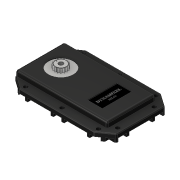
# Autodesk Inventor part: Depan
Saved by Autodesk Inventor 2019 (Build 230136000, 136)
## iProperties
Created: 2021-08-24
Part Number: Depan
Material: Generic
Document SubType Name: Modeling
Designer: user
Density: 1 g/cm^3
Appearance: Glossy - Black
Author: user
Autodesk Inventor part; units mm, degrees
(part 1 of 2)
ref_plane "YZ Plane" through (0, 0, 0) normal (1, 0, 0) x (0, 1, 0)
ref_plane "XZ Plane" through (0, 0, 0) normal (0, 1, 0) x (-1, 0, 0)
ref_plane "XY Plane" through (0, 0, 0) normal (0, 0, 1) x (1, 0, 0)
sketch "Sketch1" plane through (0, 0, 0) normal (0, 1, 0) x (-1, 0, 0)
  line L0 (30.55, -20.1) -> (-30.55, -20.1)
  line L1 (-30.55, -20.1) -> (-30.55, 20.1)
  line L2 (-30.55, 20.1) -> (30.55, 20.1)
  line L3 (30.55, 20.1) -> (30.55, -20.1)
  line L4 (30.55, -20.1) -> (-30.55, 20.1) construction
  line L5 (-30.55, -20.1) -> (30.55, 20.1) construction
  circle A0 centre (17.55, 0) radius 5
  circle A1 centre (17.55, 0) radius 14
  line L6 (-24.95, -14.5) -> (30.55, -14.5)
  line L7 (30.55, -14.5) -> (30.55, 14.5)
  line L8 (30.55, 14.5) -> (-24.95, 14.5)
  line L9 (-24.95, 14.5) -> (-24.95, -14.5)
  line L10 (-24.95, -14.5) -> (30.55, 14.5) construction
  line L11 (30.55, -14.5) -> (-24.95, 14.5) construction
  circle A2 centre (21.55, 17.3) radius 1.25
  circle A3 centre (21.55, -17.3) radius 1.25
  circle A4 centre (-0.45, 17.3) radius 1.25
  circle A5 centre (-0.45, -17.3) radius 1.25
  circle A6 centre (-22.45, 17.3) radius 1.25
  circle A7 centre (-22.45, -17.3) radius 1.25
  circle A8 centre (-27.75, -11) radius 1.25
  circle A9 centre (-27.75, 11) radius 1.25
  line L12 (30.55, 14.5) -> (22.55, 20.1)
  line L13 (-30.55, 14.5) -> (-22.55, 20.1)
  line L14 (30.55, -14.5) -> (22.55, -20.1)
  line L15 (-30.55, -14.5) -> (-22.55, -20.1)
  point P0 (0, 0)
  point P1 (2.8, 0)
  point P2 (30.55, 0)
  dimension "d0" = 61.1
  dimension "d1" = 40.2
  dimension "d2" = 10
  dimension "d3" = 13
  dimension "d4" = 28
  dimension "d5" = 55.5
  dimension "d6" = 29
  dimension "d9" = 4
  dimension "d10" = 2.8
  dimension "d13" = 34.6
  dimension "d16" = 22
  dimension "d20" = 2.8
  dimension "d23" = 22
  dimension "d24" = 11
  dimension "d25" = 8
  constraints: 32 end point, 10 centre point, 6 point on line, 5 midpoint, 4 parallel, 3 horizontal, 2 perpendicular, 1 coincident, 1 vertical, 10 other
  measures "d0" distance of L1.end L2.end
  measures "d1" distance of L0.end L1.end
  measures "d2" diameter of A0
  measures "d3" distance from line of L3 A0.centre
  measures "d4" diameter of A1
  measures "d5" distance of L8.end L7.end
  measures "d6" distance of L7.end L6.end
  measures "d9" horizontal distance of A2.centre A0.centre
  measures "d10" distance from line of L2 A2.centre
  measures "d13" distance of A2.centre A3.centre
  measures "d16" distance of A2.centre A4.centre
  measures "d20" distance from line of L1 A8.centre
  measures "d23" distance of A9.centre A8.centre
  measures "d24" vertical distance of A8.centre point (0, 0)
  measures "d25" distance of L2.end L12.end
extrude "Extrusion1" add sketch "Sketch1" against normal blind 4.6 contours L0 L15 L1 L13 L2 L12 L8 L9 L6 L14 | L6 L9 L8 L3 A1 | A1 L3 | A0 picked at (27.8833, 0)
sketch "Sketch2" plane through (0, 0, 0) normal (0, 1, 0) x (1, 0, 0)
  line L0 (-30.55, 20.1) -> (30.55, -20.1) construction
  line L1 (30.55, 20.1) -> (-30.55, -20.1) construction
  circle A0 centre (-17.55, 0) radius 1.25
  circle A1 centre (-17.55, 0) radius 14
  line L2 (24.95, 14.5) -> (-30.55, 14.5)
  line L3 (-30.55, 14.5) -> (-30.55, -14.5)
  line L4 (-30.55, -14.5) -> (24.95, -14.5)
  line L5 (24.95, -14.5) -> (24.95, 14.5)
  line L6 (24.95, 14.5) -> (-30.55, -14.5) construction
  line L7 (-30.55, 14.5) -> (24.95, -14.5) construction
  point P0 (0, 0)
  point P1 (0, 0)
  point P2 (-2.8, 0)
  point P3 (-30.55, 0)
  dimension "d33" = 2.5
  dimension "d34" = 28
  dimension "d35" = 55.5
  dimension "d36" = 29
  constraints: 16 end point, 5 midpoint, 2 centre point, 2 parallel, 1 coincident, 1 perpendicular
  measures "d33" diameter of A0
  measures "d34" diameter of A1
  measures "d35" distance of L7.end L3.end
  measures "d36" distance of L3.end L3.start
extrude "Extrusion2" add sketch "Sketch2" along normal blind 3.5 contours A1 L3 | A1 L3 L2 L5 L4 picked at (-26.6333, 0)
fillet "Fillet1" radius 1 15 edges at (30.55, -2.3, -14.5) (22.55, -2.3, -20.1) (30.55, -2.3, 14.5) (22.55, -2.3, 20.1) (-22.55, -2.3, 20.1) (-22.55, -2.3, -20.1) (24.95, 1.75, -14.5) (24.95, 1.75, 14.5) (-30.55, 1.75, 14.5) (-30.55, 1.75, -14.5) (-30.55, -2.3, -14.5) (-30.55, -2.3, 14.5) (24.95, 3.5, 0) (-2.8, 3.5, -14.5) (-2.8, 3.5, 14.5)
fillet "Fillet2" radius 0.5 17 edges at (22.5354, 0, 20.0537) (26.4659, 0, 17.3589) (30.437, 0, 14.4412) (30.55, 0, 0) (30.437, 0, -14.4412) (26.4659, 0, -17.3589) (22.5354, 0, -20.0537) (0, 0, -20.1) (-22.5354, 0, -20.0537) (-26.4659, 0, -17.3589) (-30.437, 0, -14.4412) (-30.55, 0, -13.7397) (-22.5354, 0, 20.0537) (-26.4659, 0, 17.3589) (-30.437, 0, 14.4412) (-30.55, 0, 13.7397) (0, 0, 20.1)
fillet "Fillet3" radius 2 3 edges at (-30.2571, 3.2071, 14.2071) (-30.2571, 3.2071, -14.2071) (-30.55, 3.5, 0)
sketch "Sketch4" plane through (0, 3.5, 0) normal (0, 1, 0) x (1, 0, 0)
  circle A0 centre (-17.55, 0) radius 1.25 projected
  circle A1 centre (-17.55, 0) radius 7.5
  line L0 (7.45, -9) -> (16.45, -9)
  line L1 (16.45, -9) -> (16.45, 9)
  line L2 (16.45, 9) -> (7.45, 9)
  line L3 (7.45, 9) -> (7.45, -9)
  line L4 (7.45, -9) -> (16.45, 9) construction
  line L5 (16.45, -9) -> (7.45, 9) construction
  point P0 (0, 0)
  point P1 (11.95, 0)
  dimension "d53" = 15
  dimension "d63" = 9
  dimension "d64" = 18
  dimension "d65" = 25
  constraints: 12 end point, 2 midpoint, 2 parallel, 1 centre point, 1 coincident, 1 horizontal, 1 perpendicular
  measures "d53" diameter of A1
  measures "d63" distance of L2.end L1.end
  measures "d64" distance of L1.end L0.end
  measures "d65" distance from line of L3 A1.centre
extrude "Extrusion3" cut sketch "Sketch4" against normal blind 0.5
sketch "Sketch5" plane through (-17.55, 3, 0) normal (0, 1, 0) x (1, 0, 0)
  line L0 (-1.8334, 2.6835) -> (-2.7146, 2.7146)
  line L1 (-2.7146, 2.7146) -> (-2.6835, 1.8334)
  arc A0 (-1.8334, 2.6835) -> (-2.6835, 1.8334) centre (0, 0) ccw
  line L2 (-0.667, 3.1808) -> (-1.4691, 3.5467)
  line L3 (-1.4691, 3.5467) -> (-1.7776, 2.7208)
  arc A1 (-0.667, 3.1808) -> (-1.7776, 2.7208) centre (0, 0) ccw
  arc A2 (0.6011, 3.1939) -> (-0.6011, 3.1939) centre (0, 0) ccw
  line L4 (0.6011, 3.1939) -> (0, 3.839)
  line L5 (0, 3.839) -> (-0.6011, 3.1939)
  arc A3 (0.6011, 3.1939) -> (-0.6011, 3.1939) centre (0, 0) ccw
  line L6 (1.7776, 2.7208) -> (1.4691, 3.5467)
  line L7 (1.4691, 3.5467) -> (0.667, 3.1808)
  arc A4 (1.7776, 2.7208) -> (0.667, 3.1808) centre (0, 0) ccw
  line L8 (2.6835, 1.8334) -> (2.7146, 2.7146)
  line L9 (2.7146, 2.7146) -> (1.8334, 2.6835)
  arc A5 (2.6835, 1.8334) -> (1.8334, 2.6835) centre (0, 0) ccw
  line L10 (3.1808, 0.667) -> (3.5467, 1.4691)
  line L11 (3.5467, 1.4691) -> (2.7208, 1.7776)
  arc A6 (3.1808, 0.667) -> (2.7208, 1.7776) centre (0, 0) ccw
  line L12 (3.1939, -0.6011) -> (3.839, 0)
  line L13 (3.839, 0) -> (3.1939, 0.6011)
  arc A7 (3.1939, -0.6011) -> (3.1939, 0.6011) centre (0, 0) ccw
  line L14 (2.7208, -1.7776) -> (3.5467, -1.4691)
  line L15 (3.5467, -1.4691) -> (3.1808, -0.667)
  arc A8 (2.7208, -1.7776) -> (3.1808, -0.667) centre (0, 0) ccw
  line L16 (1.8334, -2.6835) -> (2.7146, -2.7146)
  line L17 (2.7146, -2.7146) -> (2.6835, -1.8334)
  arc A9 (1.8334, -2.6835) -> (2.6835, -1.8334) centre (0, 0) ccw
  line L18 (0.667, -3.1808) -> (1.4691, -3.5467)
  line L19 (1.4691, -3.5467) -> (1.7776, -2.7208)
  arc A10 (0.667, -3.1808) -> (1.7776, -2.7208) centre (0, 0) ccw
  line L20 (-0.6011, -3.1939) -> (0, -3.839)
  line L21 (0, -3.839) -> (0.6011, -3.1939)
  arc A11 (-0.6011, -3.1939) -> (0.6011, -3.1939) centre (0, 0) ccw
  line L22 (-1.7776, -2.7208) -> (-1.4691, -3.5467)
  line L23 (-1.4691, -3.5467) -> (-0.667, -3.1808)
  arc A12 (-1.7776, -2.7208) -> (-0.667, -3.1808) centre (0, 0) ccw
  line L24 (-2.6835, -1.8334) -> (-2.7146, -2.7146)
  line L25 (-2.7146, -2.7146) -> (-1.8334, -2.6835)
  arc A13 (-2.6835, -1.8334) -> (-1.8334, -2.6835) centre (0, 0) ccw
  line L26 (-3.1808, -0.667) -> (-3.5467, -1.4691)
  line L27 (-3.5467, -1.4691) -> (-2.7208, -1.7776)
  arc A14 (-3.1808, -0.667) -> (-2.7208, -1.7776) centre (0, 0) ccw
  line L28 (-3.1939, 0.6011) -> (-3.839, 0)
  line L29 (-3.839, 0) -> (-3.1939, -0.6011)
  arc A15 (-3.1939, 0.6011) -> (-3.1939, -0.6011) centre (0, 0) ccw
  line L30 (-2.7208, 1.7776) -> (-3.5467, 1.4691)
  line L31 (-3.5467, 1.4691) -> (-3.1808, 0.667)
  arc A16 (-2.7208, 1.7776) -> (-3.1808, 0.667) centre (0, 0) ccw
  circle A17 centre (0, 0) radius 3.25
  circle A18 centre (0, 0) radius 1.25
  point P0 (17.55, 0)
  constraints: 64 end point, 34 point on circle, 19 centre point
extrude "Extrusion4" add sketch "Sketch5" along normal blind 2.5 contours A17 A1 A2 A4 A5 A6 A7 A8 A9 A10 A11 A12 A13 A14 A15 A16 A0
sketch "Sketch6" plane through (-17.55, 3, 0) normal (0, 1, 0) x (1, 0, 0)
  line L0 (-1.8334, 2.6835) -> (-2.7146, 2.7146)
  line L1 (-2.7146, 2.7146) -> (-2.6835, 1.8334)
  arc A0 (-1.8334, 2.6835) -> (-2.6835, 1.8334) centre (0, 0) ccw
  circle A1 centre (0, 0) radius 3.25
  circle A2 centre (0, 0) radius 1.25
  arc A3 (1.7776, 2.7208) -> (0.667, 3.1808) centre (0, 0) ccw
  arc A4 (-0.667, 3.1808) -> (-1.7776, 2.7208) centre (0, 0) ccw
  line L2 (-0.667, 3.1808) -> (-1.4691, 3.5467)
  line L3 (-1.4691, 3.5467) -> (-1.7776, 2.7208)
  arc A5 (0.6011, 3.1939) -> (-0.6011, 3.1939) centre (0, 0) ccw
  line L4 (0.6011, 3.1939) -> (0, 3.839)
  line L5 (0, 3.839) -> (-0.6011, 3.1939)
  line L6 (1.7776, 2.7208) -> (1.4691, 3.5467)
  line L7 (1.4691, 3.5467) -> (0.667, 3.1808)
  arc A6 (0.6011, 3.1939) -> (-0.6011, 3.1939) centre (0, 0) ccw
  arc A7 (3.1808, 0.667) -> (2.7208, 1.7776) centre (0, 0) ccw
  line L8 (3.1808, 0.667) -> (3.5467, 1.4691)
  line L9 (3.5467, 1.4691) -> (2.7208, 1.7776)
  arc A8 (2.6835, 1.8334) -> (1.8334, 2.6835) centre (0, 0) ccw
  line L10 (2.7146, 2.7146) -> (1.8334, 2.6835)
  line L11 (2.6835, 1.8334) -> (2.7146, 2.7146)
  arc A9 (2.7208, -1.7776) -> (3.1808, -0.667) centre (0, 0) ccw
  line L12 (2.7208, -1.7776) -> (3.5467, -1.4691)
  line L13 (3.5467, -1.4691) -> (3.1808, -0.667)
  arc A10 (3.1939, -0.6011) -> (3.1939, 0.6011) centre (0, 0) ccw
  line L14 (3.1939, -0.6011) -> (3.839, 0)
  line L15 (3.839, 0) -> (3.1939, 0.6011)
  arc A11 (-2.6835, -1.8334) -> (-1.8334, -2.6835) centre (0, 0) ccw
  line L16 (-2.6835, -1.8334) -> (-2.7146, -2.7146)
  line L17 (-2.7146, -2.7146) -> (-1.8334, -2.6835)
  arc A12 (-1.7776, -2.7208) -> (-0.667, -3.1808) centre (0, 0) ccw
  line L18 (-1.7776, -2.7208) -> (-1.4691, -3.5467)
  arc A13 (-0.6011, -3.1939) -> (0.6011, -3.1939) centre (0, 0) ccw
  line L19 (0.667, -3.1808) -> (1.4691, -3.5467)
  line L20 (2.7146, -2.7146) -> (2.6835, -1.8334)
  line L21 (1.8334, -2.6835) -> (2.7146, -2.7146)
  line L22 (1.4691, -3.5467) -> (1.7776, -2.7208)
  arc A14 (1.8334, -2.6835) -> (2.6835, -1.8334) centre (0, 0) ccw
  line L23 (-1.4691, -3.5467) -> (-0.667, -3.1808)
  line L24 (0, -3.839) -> (0.6011, -3.1939)
  line L25 (-0.6011, -3.1939) -> (0, -3.839)
  arc A15 (0.667, -3.1808) -> (1.7776, -2.7208) centre (0, 0) ccw
  line L26 (-3.5467, 1.4691) -> (-3.1808, 0.667)
  arc A16 (-2.7208, 1.7776) -> (-3.1808, 0.667) centre (0, 0) ccw
  line L27 (-2.7208, 1.7776) -> (-3.5467, 1.4691)
  arc A17 (-3.1939, 0.6011) -> (-3.1939, -0.6011) centre (0, 0) ccw
  arc A18 (-3.1808, -0.667) -> (-2.7208, -1.7776) centre (0, 0) ccw
  line L28 (-3.1939, 0.6011) -> (-3.839, 0)
  line L29 (-3.839, 0) -> (-3.1939, -0.6011)
  line L30 (-3.5467, -1.4691) -> (-2.7208, -1.7776)
  line L31 (-3.1808, -0.667) -> (-3.5467, -1.4691)
  point P0 (17.55, 0)
  constraints: 64 end point, 34 point on circle, 19 centre point
extrude "Extrusion5" add sketch "Sketch6" along normal blind 2.4 contours A0 L1 L0 | L3 L2 A1 | A1 L26 L27 | L5 L4 A1 | A1 L29 L28 | L7 L6 A1 | A1 L30 L31 | L10 L11 A1 | A1 L17 L16 | L9 L8 A1 | A1 L23 L18 | L15 L14 A1 | A1 L24 L25 | A1 L22 L19 | L13 L12 A1 | A1 L20 L21
chamfer "Chamfer1" distance 0.1 angle 45 2 edges at (-20.8, 5.5, 0) (-18.8, 5.5, 0)
sketch "Sketch7" plane through (0, -4.6, 0) normal (0, -1, 0) x (1, 0, 0)
  line L0 (-22.2348, -20.1) -> (22.2348, -20.1) projected
  circle A0 centre (-21.55, -17.3) radius 1.25 projected
  line L1 (-21.55, -14.4132) -> (-19.05, -15.8566)
  line L2 (-19.05, -15.8566) -> (-19.05, -18.7434)
  line L3 (-19.05, -18.7434) -> (-21.55, -20.1868)
  line L4 (-21.55, -20.1868) -> (-24.05, -18.7434)
  line L5 (-24.05, -18.7434) -> (-24.05, -15.8566)
  line L6 (-24.05, -15.8566) -> (-21.55, -14.4132)
  line L7 (-17.55, -19.6094) -> (-17.55, -14.9906)
  line L8 (-17.55, -14.9906) -> (-21.55, -12.6812)
  line L9 (-21.55, -12.6812) -> (-25.55, -14.9906)
  line L10 (-25.55, -14.9906) -> (-25.55, -19.6094)
  line L11 (-25.55, -19.6094) -> (-21.55, -21.9188)
  line L12 (-21.55, -21.9188) -> (-17.55, -19.6094)
  circle A1 centre (27.75, -11) radius 1.25 projected
  line L13 (24.8632, -11) -> (26.3066, -8.5)
  line L14 (26.3066, -8.5) -> (29.1934, -8.5)
  line L15 (29.1934, -8.5) -> (30.6368, -11)
  line L16 (30.6368, -11) -> (29.1934, -13.5)
  line L17 (29.1934, -13.5) -> (26.3066, -13.5)
  line L18 (26.3066, -13.5) -> (24.8632, -11)
  line L19 (23.1312, -11) -> (25.4406, -7)
  line L20 (25.4406, -7) -> (30.0594, -7)
  line L21 (30.0594, -7) -> (32.3688, -11)
  line L22 (32.3688, -11) -> (30.0594, -15)
  line L23 (30.0594, -15) -> (25.4406, -15)
  line L24 (25.4406, -15) -> (23.1312, -11)
  line L25 (0.45, -12.6812) -> (-3.55, -14.9906)
  line L26 (-2.05, -15.8566) -> (0.45, -14.4132)
  line L27 (4.45, -14.9906) -> (0.45, -12.6812)
  line L28 (0.45, -14.4132) -> (2.95, -15.8566)
  line L29 (-2.05, -18.7434) -> (-2.05, -15.8566)
  line L30 (-3.55, -14.9906) -> (-3.55, -19.6094)
  line L31 (-3.55, -19.6094) -> (0.45, -21.9188)
  line L32 (0.45, -20.1868) -> (-2.05, -18.7434)
  line L33 (2.95, -15.8566) -> (2.95, -18.7434)
  line L34 (4.45, -19.6094) -> (4.45, -14.9906)
  line L35 (2.95, -18.7434) -> (0.45, -20.1868)
  line L36 (0.45, -21.9188) -> (4.45, -19.6094)
  line L37 (22.45, -12.6812) -> (18.45, -14.9906)
  line L38 (19.95, -15.8566) -> (22.45, -14.4132)
  line L39 (26.45, -14.9906) -> (22.45, -12.6812)
  line L40 (22.45, -14.4132) -> (24.95, -15.8566)
  line L41 (19.95, -18.7434) -> (19.95, -15.8566)
  line L42 (18.45, -14.9906) -> (18.45, -19.6094)
  line L43 (18.45, -19.6094) -> (22.45, -21.9188)
  line L44 (22.45, -20.1868) -> (19.95, -18.7434)
  line L45 (24.95, -15.8566) -> (24.95, -18.7434)
  line L46 (26.45, -19.6094) -> (26.45, -14.9906)
  line L47 (24.95, -18.7434) -> (22.45, -20.1868)
  line L48 (22.45, -21.9188) -> (26.45, -19.6094)
  line L49 (30.55, 13.9793) -> (30.55, -13.9793) projected
  line L50 (30.55, 0) -> (-30.55, 0)
  line L51 (-30.55, 13.9793) -> (-30.55, -13.9793) projected
  line L52 (22.2348, -20.1) -> (-22.2348, -20.1) projected
  line L53 (4.45, -14.9906) -> (18.45, -14.9906)
  line L54 (18.45, -14.9906) -> (18.45, -20.1)
  line L55 (18.45, -20.1) -> (4.45, -20.1)
  line L56 (4.45, -20.1) -> (4.45, -14.9906)
  line L57 (-3.55, -14.9906) -> (-17.55, -14.9906)
  line L58 (-17.55, -14.9906) -> (-17.55, -20.1)
  line L59 (-17.55, -20.1) -> (-3.55, -20.1)
  line L60 (-3.55, -20.1) -> (-3.55, -14.9906)
  line L61 (-22.8082, -19.9192) -> (-29.9795, -14.8994) projected
  line L62 (-25.55, -14.9906) -> (-25.55, -18)
  line L63 (-25.55, -18) -> (-29.8789, -14.9698)
  line L64 (-24.05, -18.7434) -> (-19.05, -18.7434)
  line L65 (-19.05, -18.7434) -> (-19.05, -20.1)
  line L66 (-19.05, -20.1) -> (-24.05, -20.1)
  line L67 (-24.05, -20.1) -> (-24.05, -18.7434)
  line L68 (2.95, -18.7434) -> (-2.05, -18.7434)
  line L69 (-2.05, -18.7434) -> (-2.05, -20.1)
  line L70 (-2.05, -20.1) -> (2.95, -20.1)
  line L71 (2.95, -20.1) -> (2.95, -18.7434)
  line L72 (19.95, -18.7434) -> (24.95, -18.7434)
  line L73 (24.95, -18.7434) -> (24.95, -20.1)
  line L74 (24.95, -20.1) -> (19.95, -20.1)
  line L75 (19.95, -20.1) -> (19.95, -18.7434)
  line L76 (29.1934, -13.5) -> (30.55, -13.5)
  line L77 (30.55, -13.5) -> (30.55, -8.5)
  line L78 (30.55, -8.5) -> (29.1934, -8.5)
  line L79 (29.1934, -8.5) -> (29.1934, -13.5)
  line L80 (26.45, -15) -> (30.2607, -15)
  line L81 (30.2607, -15) -> (30.2607, -17.4093)
  line L82 (30.2607, -17.4093) -> (26.45, -17.4093)
  line L83 (26.45, -17.4093) -> (26.45, -15)
  line L84 (25.4406, -7) -> (30.55, -7)
  line L85 (30.55, -7) -> (30.55, 0)
  line L86 (30.55, 0) -> (25.4406, 0)
  line L87 (25.4406, 0) -> (25.4406, -7)
  line L88 (23.95, -14.5) -> (-28.55, -14.5) projected
  line L89 (18.45, -20.1) -> (4.45, -20.1)
  line L90 (4.45, -20.1) -> (4.45, -14.5)
  line L91 (4.45, -14.5) -> (18.45, -14.5)
  line L92 (18.45, -14.5) -> (18.45, -20.1)
  line L93 (-17.55, -20.1) -> (-3.55, -20.1)
  line L94 (-3.55, -20.1) -> (-3.55, -14.5)
  line L95 (-3.55, -14.5) -> (-17.55, -14.5)
  line L96 (-17.55, -14.5) -> (-17.55, -20.1)
  line L97 (-25.55, -18) -> (-25.55, -14.5)
  line L98 (-29.55, -14.5) -> (23.95, -14.5) projected
  line L99 (-25.55, -14.5) -> (-29.55, -14.5)
  line L100 (-29.55, -14.5) -> (-29.8789, -14.9698)
  line L101 (-29.8789, -14.9698) -> (-25.55, -18)
  line L102 (-30.55, -11.25) -> (-30.55, 11.25)
  line L103 (-22.2348, 20.1) -> (22.2348, 20.1)
  circle A2 centre (-21.55, 17.3) radius 1.25
  line L104 (-21.55, 14.4132) -> (-19.05, 15.8566)
  line L105 (-19.05, 15.8566) -> (-19.05, 18.7434)
  line L106 (-19.05, 18.7434) -> (-21.55, 20.1868)
  line L107 (-21.55, 20.1868) -> (-24.05, 18.7434)
  line L108 (-24.05, 18.7434) -> (-24.05, 15.8566)
  line L109 (-24.05, 15.8566) -> (-21.55, 14.4132)
  line L110 (-17.55, 19.6094) -> (-17.55, 14.9906)
  line L111 (-17.55, 14.9906) -> (-21.55, 12.6812)
  line L112 (-21.55, 12.6812) -> (-25.55, 14.9906)
  line L113 (-25.55, 14.9906) -> (-25.55, 19.6094)
  line L114 (-25.55, 19.6094) -> (-21.55, 21.9188)
  line L115 (-21.55, 21.9188) -> (-17.55, 19.6094)
  circle A3 centre (27.75, 11) radius 1.25
  line L116 (24.8632, 11) -> (26.3066, 8.5)
  line L117 (26.3066, 8.5) -> (29.1934, 8.5)
  line L118 (29.1934, 8.5) -> (30.6368, 11)
  line L119 (30.6368, 11) -> (29.1934, 13.5)
  line L120 (29.1934, 13.5) -> (26.3066, 13.5)
  line L121 (26.3066, 13.5) -> (24.8632, 11)
  line L122 (23.1312, 11) -> (25.4406, 7)
  line L123 (25.4406, 7) -> (30.0594, 7)
  line L124 (30.0594, 7) -> (32.3688, 11)
  line L125 (32.3688, 11) -> (30.0594, 15)
  line L126 (30.0594, 15) -> (25.4406, 15)
  line L127 (25.4406, 15) -> (23.1312, 11)
  line L128 (0.45, 12.6812) -> (-3.55, 14.9906)
  line L129 (-2.05, 15.8566) -> (0.45, 14.4132)
  line L130 (4.45, 14.9906) -> (0.45, 12.6812)
  line L131 (0.45, 14.4132) -> (2.95, 15.8566)
  line L132 (-2.05, 18.7434) -> (-2.05, 15.8566)
  line L133 (-3.55, 14.9906) -> (-3.55, 19.6094)
  line L134 (-3.55, 19.6094) -> (0.45, 21.9188)
  line L135 (0.45, 20.1868) -> (-2.05, 18.7434)
  line L136 (2.95, 15.8566) -> (2.95, 18.7434)
  line L137 (4.45, 19.6094) -> (4.45, 14.9906)
  line L138 (2.95, 18.7434) -> (0.45, 20.1868)
  line L139 (0.45, 21.9188) -> (4.45, 19.6094)
  line L140 (22.45, 12.6812) -> (18.45, 14.9906)
  line L141 (19.95, 15.8566) -> (22.45, 14.4132)
  line L142 (26.45, 14.9906) -> (22.45, 12.6812)
  line L143 (22.45, 14.4132) -> (24.95, 15.8566)
  line L144 (19.95, 18.7434) -> (19.95, 15.8566)
  line L145 (18.45, 14.9906) -> (18.45, 19.6094)
  line L146 (18.45, 19.6094) -> (22.45, 21.9188)
  line L147 (22.45, 20.1868) -> (19.95, 18.7434)
  line L148 (24.95, 15.8566) -> (24.95, 18.7434)
  line L149 (26.45, 19.6094) -> (26.45, 14.9906)
  line L150 (24.95, 18.7434) -> (22.45, 20.1868)
  line L151 (22.45, 21.9188) -> (26.45, 19.6094)
  line L152 (30.55, -13.9793) -> (30.55, 13.9793)
  line L153 (22.2348, 20.1) -> (-22.2348, 20.1)
  line L154 (4.45, 14.9906) -> (18.45, 14.9906)
  line L155 (18.45, 14.9906) -> (18.45, 20.1)
  line L156 (18.45, 20.1) -> (4.45, 20.1)
  line L157 (4.45, 20.1) -> (4.45, 14.9906)
  line L158 (-3.55, 14.9906) -> (-17.55, 14.9906)
  line L159 (-17.55, 14.9906) -> (-17.55, 20.1)
  line L160 (-17.55, 20.1) -> (-3.55, 20.1)
  line L161 (-3.55, 20.1) -> (-3.55, 14.9906)
  line L162 (-22.8082, 19.9192) -> (-29.9795, 14.8994)
  line L163 (-25.55, 14.9906) -> (-25.55, 18)
  line L164 (-25.55, 18) -> (-29.8789, 14.9698)
  line L165 (-24.05, 18.7434) -> (-19.05, 18.7434)
  line L166 (-19.05, 18.7434) -> (-19.05, 20.1)
  line L167 (-19.05, 20.1) -> (-24.05, 20.1)
  line L168 (-24.05, 20.1) -> (-24.05, 18.7434)
  line L169 (2.95, 18.7434) -> (-2.05, 18.7434)
  line L170 (-2.05, 18.7434) -> (-2.05, 20.1)
  line L171 (-2.05, 20.1) -> (2.95, 20.1)
  line L172 (2.95, 20.1) -> (2.95, 18.7434)
  line L173 (19.95, 18.7434) -> (24.95, 18.7434)
  line L174 (24.95, 18.7434) -> (24.95, 20.1)
  line L175 (24.95, 20.1) -> (19.95, 20.1)
  line L176 (19.95, 20.1) -> (19.95, 18.7434)
  line L177 (29.1934, 13.5) -> (30.55, 13.5)
  line L178 (30.55, 13.5) -> (30.55, 8.5)
  line L179 (30.55, 8.5) -> (29.1934, 8.5)
  line L180 (29.1934, 8.5) -> (29.1934, 13.5)
  line L181 (26.45, 15) -> (30.2607, 15)
  line L182 (30.2607, 15) -> (30.2607, 17.4093)
  line L183 (30.2607, 17.4093) -> (26.45, 17.4093)
  line L184 (26.45, 17.4093) -> (26.45, 15)
  line L185 (25.4406, 7) -> (30.55, 7)
  line L186 (25.4406, 0) -> (25.4406, 7)
  line L187 (23.95, 14.5) -> (-28.55, 14.5)
  line L188 (18.45, 20.1) -> (4.45, 20.1)
  line L189 (4.45, 20.1) -> (4.45, 14.5)
  line L190 (4.45, 14.5) -> (18.45, 14.5)
  line L191 (18.45, 14.5) -> (18.45, 20.1)
  line L192 (-17.55, 20.1) -> (-3.55, 20.1)
  line L193 (-3.55, 20.1) -> (-3.55, 14.5)
  line L194 (-3.55, 14.5) -> (-17.55, 14.5)
  line L195 (-17.55, 14.5) -> (-17.55, 20.1)
  line L196 (-25.55, 18) -> (-25.55, 14.5)
  line L197 (-29.55, 14.5) -> (23.95, 14.5)
  line L198 (-25.55, 14.5) -> (-29.55, 14.5)
  line L199 (-29.55, 14.5) -> (-29.8789, 14.9698)
  line L200 (-29.8789, 14.9698) -> (-25.55, 18)
  line L201 (25.4406, 7) -> (30.55, 7)
  line L202 (30.55, 7) -> (30.55, 0)
  line L203 (30.55, 0) -> (25.4406, 0)
  line L204 (25.4406, 0) -> (25.4406, 7)
  line L205 (-29.8789, 14.9698) -> (-30.55, 14.5)
  line L206 (-22.8082, 19.9192) -> (-30.1235, 14.7986) projected
  arc A4 (-29.55, 14.5) -> (-29.6927, 14.4898) centre (-29.55, 13.5) ccw projected
  line L207 (-30.55, 14.5) -> (-29.55, 14.5)
  line L208 (-29.55, 14.5) -> (-29.8789, 14.9698)
  arc A5 (-29.6927, -14.4898) -> (-29.55, -14.5) centre (-29.55, -13.5) ccw projected
  line L209 (-29.55, -14.5) -> (-30.55, -14.5)
  line L210 (-30.55, -14.5) -> (-29.8789, -14.9698)
  line L211 (-30.1235, -14.7986) -> (-22.8082, -19.9192) projected
  line L212 (-29.8789, -14.9698) -> (-29.55, -14.5)
  point P0 (0, 0)
  point P1 (0.45, -17.3)
  point P2 (0.45, -17.3)
  point P3 (-0.2348, -20.1)
  point P4 (22.45, -17.3)
  point P5 (22.45, -17.3)
  point P6 (21.7652, -20.1)
  point P7 (0.45, 17.3)
  point P8 (0.45, 17.3)
  point P9 (-0.2348, 20.1)
  point P10 (22.45, 17.3)
  point P11 (22.45, 17.3)
  point P12 (21.7652, 20.1)
  dimension "d66" = 5
  dimension "d67" = 1.5
  dimension "d68" = 5
  dimension "d69" = 1.5
  dimension "d72" = 22
  dimension "d78" = 22.5
  constraints: 408 end point, 99 symmetric about line, 30 point on line, 22 parallel, 15 perpendicular, 14 horizontal, 8 coincident, 4 collinear, 2 centre point, 2 midpoint, 2 tangent, 92 other
  measures "d66" distance between parallel lines of L5 L2
  measures "d67" distance between parallel lines of L2 L7
  measures "d68" distance between parallel lines of L14 L17
  measures "d69" distance between parallel lines of L18 L24
  measures "d72" distance of L9.end L25.end
  measures "d78" distance of L102.start L102.end
extrude "Extrusion6" cut sketch "Sketch7" against normal blind 2 contours L58 L7 L57 L30 L60 L0 | L0 L3 L65 | L96 L88 L94 L57 | L69 L32 L0 | L3 L4 L0 | L0 L4 L64 L3 | L64 L5 L6 L88 L1 L2 | L32 L68 L35 L0 | L0 L35 L32 | L29 L26 L88 L28 L33 L68 | L0 L66 L67 L4 | L61 L100 L98 L88 L97 L10 | L88 L6 L1 | L35 L71 L0 | L56 L34 L53 L42 L54 L0 | L26 L28 L88 | L61 L210 L209 L100 | L90 L88 L92 L53 | L75 L44 L74 L0 | L72 L47 L74 L44 | L41 L38 L88 L40 L45 L72 | L38 L40 L88 | L74 L47 L44 | L73 L74 L47 | L46 L23 L80 L81 L82 | L87 L50 L49 L84 L20 | L186 L123 L185 L49 L50 | L126 L149 L183 L182 L181 | L154 L137 L157 L103 L155 L145 | L191 L187 L189 L154 | L187 L143 L141 | L141 L144 L173 L148 L143 L187 | L176 L103 L175 L147 | L147 L175 L150 L173 | L187 L129 L132 L169 L136 L131 | L131 L129 L187 | L147 L150 L175 | L150 L175 L174 | L172 L138 L103 | L158 L110 L159 L103 L161 L133 | L193 L187 L195 L158 | L169 L135 L103 L138 | L103 L135 L138 | L170 L103 L135 | L187 L109 L108 L165 L105 L104 | L104 L109 L187 | L166 L106 L103 | L106 L165 L107 L103 | L103 L107 L106 | L196 L187 L197 L199 L162 L113 | L107 L168 L167 L103 | L199 L207 L205 L162 | L13 L14 L79 L17 L18 | L78 L49 L15 | L15 L49 L16 L79 | L16 L49 L76 | L15 L16 L49 | L49 L119 L177 | L119 L118 L49 | L49 L118 L180 L119 | L180 L117 L116 L121 L120 | L49 L179 L118
thread "Thread1" size "M2.5x0.45" class "6H" standard "ANSI Metric M Profile" full length
fillet "Fillet4" radius 2 2 edges at (-30.4038, -3.6, -14.5) (-30.4038, -3.6, 14.5)
sketch "Sketch9" plane through (0, 0, 0) normal (0, 0, 1) x (1, 0, 0)
  line L0 (-20.7, 5.5) -> (-14.4, 5.5) projected
  arc A0 (-20.35, 5.5) -> (-19.85, 5.5) centre (-20.1, 5.5) ccw
  line L1 (-19.85, 5.5) -> (-20.35, 5.5)
  point P0 (0, 0)
  dimension "d86" = 0.6
  constraints: 3 point on line, 2 end point, 2 point on circle, 1 centre point, 1 collinear
  measures "d86" distance of A0.centre L0.start
revolve "Revolution1" cut sketch "Sketch9" angle 360 about axis through (-19.85, 5.5, 0) along (-1, 0, 0)
sketch "Sketch10" plane through (0, 3, 0) normal (0, 1, 0) x (1, 0, 0)
  line L0 (16.45, -9) -> (7.45, -9) projected
  line L1 (16.45, 9) -> (16.45, -9) projected
  line L2 (7.45, 9) -> (16.45, 9) projected
  line L3 (7.45, -9) -> (7.45, 9) projected
  line L4 (3.1428, -4.3466) -> (3.1428, 4.5307) construction
  line L5 (3.1428, 4.5307) -> (21.1886, 4.5307) construction
  line L6 (21.1886, 4.5307) -> (21.1886, -4.3466) construction
  line L7 (21.1886, -4.3466) -> (3.1428, -4.3466) construction
  line L8 (11.793, -7.0811) -> (11.7316, -6.9201)
  spline S0 degree 2 poles (11.7316, -6.9201) (11.725, -6.9035) (11.7018, -6.8803) (11.6785, -6.8803) knots 0 0 0 1 2 2 2
  line L9 (11.6785, -6.8803) -> (10.5834, -6.8803)
  spline S1 degree 2 poles (10.5834, -6.8803) (10.5618, -6.8803) (10.5403, -6.9035) (10.5336, -6.9201) knots 0 0 0 1 2 2 2
  line L10 (10.5336, -6.9201) -> (10.4722, -7.0811)
  line L11 (10.4722, -7.0811) -> (10.3826, -7.0811)
  line L12 (10.3826, -7.0811) -> (10.3826, -6.3327)
  spline S2 degree 2 poles (10.3826, -6.3327) (10.3826, -6.2498) (10.4108, -6.0689) (10.4772, -5.8914) (10.5884, -5.7304) (10.756, -5.606) (10.9833, -5.533) (11.1343, -5.533) knots 0 0 0 1 2 3 4 5 6 6 6
  spline S3 degree 2 poles (11.1343, -5.533) (11.3268, -5.533) (11.6088, -5.6591) (11.793, -5.8781) (11.8826, -6.1734) (11.8826, -6.3443) knots 0 0 0 1 2 3 4 4 4
  line L13 (11.8826, -6.3443) -> (11.8826, -7.0811)
  line L14 (11.8826, -7.0811) -> (11.793, -7.0811)
  spline S4 degree 2 poles (11.7084, -6.3278) (11.7084, -6.2182) (11.6354, -6.0573) (11.496, -5.9544) (11.2936, -5.9046) (11.1658, -5.9046) knots 0 0 0 1 2 3 4 4 4
  spline S5 degree 2 poles (11.1658, -5.9046) (11.0231, -5.9046) (10.7991, -5.971) (10.6415, -6.0955) (10.5568, -6.273) (10.5568, -6.3825) knots 0 0 0 1 2 3 4 4 4
  line L15 (10.5568, -6.3825) -> (10.5568, -6.5352)
  line L16 (10.5568, -6.5352) -> (11.7084, -6.5352)
  line L17 (11.7084, -6.5352) -> (11.7084, -6.3278)
  line L18 (11.793, -5.0567) -> (11.7316, -4.8842)
  spline S6 degree 2 poles (11.7316, -4.8842) (11.725, -4.8659) (11.7018, -4.8443) (11.6785, -4.8443) knots 0 0 0 1 2 2 2
  line L19 (11.6785, -4.8443) -> (11.3185, -4.8443)
  line L20 (11.3185, -4.8443) -> (10.5734, -5.2675)
  spline S7 degree 2 poles (10.5734, -5.2675) (10.5568, -5.2758) (10.527, -5.3007) (10.5187, -5.3206) knots 0 0 0 1 2 2 2
  line L21 (10.5187, -5.3206) -> (10.4722, -5.4367)
  line L22 (10.4722, -5.4367) -> (10.3826, -5.4367)
  line L23 (10.3826, -5.4367) -> (10.3826, -4.7531)
  line L24 (10.3826, -4.7531) -> (10.4722, -4.7531)
  line L25 (10.4722, -4.7531) -> (10.5336, -4.924)
  line L26 (10.5336, -4.924) -> (10.9916, -4.6552)
  line L27 (10.9916, -4.6552) -> (11.121, -4.5988)
  line L28 (11.121, -4.5988) -> (11.121, -4.5822)
  line L29 (11.121, -4.5822) -> (10.5419, -4.2536)
  line L30 (10.5419, -4.2536) -> (10.4722, -4.4229)
  line L31 (10.4722, -4.4229) -> (10.3826, -4.4229)
  line L32 (10.3826, -4.4229) -> (10.3826, -3.8986)
  line L33 (10.3826, -3.8986) -> (10.4722, -3.8986)
  line L34 (10.4722, -3.8986) -> (10.5253, -4.013)
  spline S8 degree 2 poles (10.5253, -4.013) (10.532, -4.0296) (10.5635, -4.0578) (10.5784, -4.0678) knots 0 0 0 1 2 2 2
  line L35 (10.5784, -4.0678) -> (11.3118, -4.4976)
  line L36 (11.3118, -4.4976) -> (11.6785, -4.4976)
  spline S9 degree 2 poles (11.6785, -4.4976) (11.7018, -4.4976) (11.725, -4.476) (11.7316, -4.4577) knots 0 0 0 1 2 2 2
  line L37 (11.7316, -4.4577) -> (11.793, -4.2852)
  line L38 (11.793, -4.2852) -> (11.8826, -4.2852)
  line L39 (11.8826, -4.2852) -> (11.8826, -5.0567)
  line L40 (11.8826, -5.0567) -> (11.793, -5.0567)
  line L41 (10.8904, -3.3012) -> (10.7526, -3.3825)
  line L42 (10.7526, -3.3825) -> (10.7526, -3.3991)
  line L43 (10.7526, -3.3991) -> (11.6719, -3.3991)
  spline S10 degree 2 poles (11.6719, -3.3991) (11.6951, -3.3991) (11.7167, -3.3759) (11.7233, -3.3593) knots 0 0 0 1 2 2 2
  line L44 (11.7233, -3.3593) -> (11.793, -3.2016)
  line L45 (11.793, -3.2016) -> (11.8826, -3.2016)
  line L46 (11.8826, -3.2016) -> (11.8826, -3.7973)
  line L47 (11.8826, -3.7973) -> (11.793, -3.7973)
  line L48 (11.793, -3.7973) -> (11.7233, -3.6364)
  spline S11 degree 2 poles (11.7233, -3.6364) (11.7167, -3.6198) (11.6951, -3.5966) (11.6719, -3.5966) knots 0 0 0 1 2 2 2
  line L49 (11.6719, -3.5966) -> (10.5834, -3.5966)
  spline S12 degree 2 poles (10.5834, -3.5966) (10.5635, -3.5966) (10.5403, -3.6198) (10.5353, -3.6364) knots 0 0 0 1 2 2 2
  line L50 (10.5353, -3.6364) -> (10.4722, -3.804)
  line L51 (10.4722, -3.804) -> (10.3826, -3.804)
  line L52 (10.3826, -3.804) -> (10.3826, -3.263)
  line L53 (10.3826, -3.263) -> (11.2886, -2.6325)
  line L54 (11.2886, -2.6325) -> (11.423, -2.5512)
  line L55 (11.423, -2.5512) -> (11.423, -2.5346)
  line L56 (11.423, -2.5346) -> (10.59, -2.5346)
  spline S13 degree 2 poles (10.59, -2.5346) (10.5685, -2.5346) (10.5502, -2.5562) (10.5419, -2.5761) knots 0 0 0 1 2 2 2
  line L57 (10.5419, -2.5761) -> (10.4722, -2.7354)
  line L58 (10.4722, -2.7354) -> (10.3826, -2.7354)
  line L59 (10.3826, -2.7354) -> (10.3826, -2.138)
  line L60 (10.3826, -2.138) -> (10.4722, -2.138)
  line L61 (10.4722, -2.138) -> (10.5419, -2.299)
  spline S14 degree 2 poles (10.5419, -2.299) (10.5469, -2.3139) (10.5685, -2.3388) (10.59, -2.3388) knots 0 0 0 1 2 2 2
  line L62 (10.59, -2.3388) -> (11.6503, -2.3388)
  line L63 (11.6503, -2.3388) -> (11.8926, -2.372)
  line L64 (11.8926, -2.372) -> (11.8926, -2.601)
  line L65 (11.8926, -2.601) -> (10.8904, -3.3012)
  line L66 (11.793, -2.0849) -> (11.7432, -1.9771)
  spline S15 degree 2 poles (11.7432, -1.9771) (11.7266, -1.9389) (11.6852, -1.9223) knots 0 0 0 1 1 1
  line L67 (11.6852, -1.9223) -> (10.6099, -1.4959)
  line L68 (10.6099, -1.4959) -> (10.3594, -1.3698)
  line L69 (10.3594, -1.3698) -> (10.3594, -1.1259)
  line L70 (10.3594, -1.1259) -> (11.6901, -0.6132)
  spline S16 degree 2 poles (11.6901, -0.6132) (11.7084, -0.6049) (11.7399, -0.58) (11.7466, -0.5634) knots 0 0 0 1 2 2 2
  line L71 (11.7466, -0.5634) -> (11.793, -0.4505)
  line L72 (11.793, -0.4505) -> (11.8826, -0.4505)
  line L73 (11.8826, -0.4505) -> (11.8826, -1.1309)
  line L74 (11.8826, -1.1309) -> (11.793, -1.1309)
  line L75 (11.793, -1.1309) -> (11.73, -0.955)
  line L76 (11.73, -0.955) -> (11.4031, -1.0861)
  line L77 (11.4031, -1.0861) -> (11.4031, -1.612)
  line L78 (11.4031, -1.612) -> (11.7233, -1.7365)
  line L79 (11.7233, -1.7365) -> (11.793, -1.5589)
  line L80 (11.793, -1.5589) -> (11.8826, -1.5589)
  line L81 (11.8826, -1.5589) -> (11.8826, -2.0849)
  line L82 (11.8826, -2.0849) -> (11.793, -2.0849)
  line L83 (11.2338, -1.1524) -> (10.8671, -1.2951)
  line L84 (10.8671, -1.2951) -> (10.7261, -1.3366)
  line L85 (10.7261, -1.3366) -> (10.7261, -1.3549)
  line L86 (10.7261, -1.3549) -> (11.2338, -1.5457)
  line L87 (11.2338, -1.5457) -> (11.2338, -1.1524)
  line L88 (11.793, -0.3742) -> (11.7233, -0.2133)
  spline S17 degree 2 poles (11.7233, -0.2133) (11.7167, -0.1967) (11.6951, -0.1734) (11.6719, -0.1734) knots 0 0 0 1 2 2 2
  line L89 (11.6719, -0.1734) -> (10.5834, -0.1734)
  spline S18 degree 2 poles (10.5834, -0.1734) (10.5618, -0.1734) (10.5386, -0.1967) (10.5336, -0.2133) knots 0 0 0 1 2 2 2
  line L90 (10.5336, -0.2133) -> (10.4722, -0.3742)
  line L91 (10.4722, -0.3742) -> (10.3826, -0.3742)
  line L92 (10.3826, -0.3742) -> (10.3826, 0.2928)
  line L93 (10.3826, 0.2928) -> (11.2372, 0.5898)
  line L94 (11.2372, 0.5898) -> (11.4197, 0.6413)
  line L95 (11.4197, 0.6413) -> (11.4197, 0.6579)
  line L96 (11.4197, 0.6579) -> (10.3826, 1.0096)
  line L97 (10.3826, 1.0096) -> (10.3826, 1.6667)
  line L98 (10.3826, 1.6667) -> (10.4722, 1.6667)
  line L99 (10.4722, 1.6667) -> (10.5336, 1.5091)
  spline S19 degree 2 poles (10.5336, 1.5091) (10.5403, 1.4925) (10.5618, 1.4659) (10.5834, 1.4659) knots 0 0 0 1 2 2 2
  line L100 (10.5834, 1.4659) -> (11.6785, 1.4659)
  spline S20 degree 2 poles (11.6785, 1.4659) (11.7018, 1.4659) (11.725, 1.4908) (11.7316, 1.5091) knots 0 0 0 1 2 2 2
  line L101 (11.7316, 1.5091) -> (11.793, 1.6667)
  line L102 (11.793, 1.6667) -> (11.8826, 1.6667)
  line L103 (11.8826, 1.6667) -> (11.8826, 0.9234)
  line L104 (11.8826, 0.9234) -> (11.793, 0.9234)
  line L105 (11.793, 0.9234) -> (11.7316, 1.0826)
  spline S21 degree 2 poles (11.7316, 1.0826) (11.7233, 1.0992) (11.7018, 1.1241) (11.6785, 1.1241) knots 0 0 0 1 2 2 2
  line L106 (11.6785, 1.1241) -> (10.6348, 1.1241)
  line L107 (10.6348, 1.1241) -> (10.6348, 1.1042)
  line L108 (10.6348, 1.1042) -> (10.7974, 1.0528)
  line L109 (10.7974, 1.0528) -> (11.6503, 0.7541)
  line L110 (11.6503, 0.7541) -> (11.8826, 0.6545)
  line L111 (11.8826, 0.6545) -> (11.8826, 0.4654)
  line L112 (11.8826, 0.4654) -> (10.7974, 0.0887)
  line L113 (10.7974, 0.0887) -> (10.6332, 0.0389)
  line L114 (10.6332, 0.0389) -> (10.6332, 0.019)
  line L115 (10.6332, 0.019) -> (11.6719, 0.019)
  spline S22 degree 2 poles (11.6719, 0.019) (11.6951, 0.019) (11.7167, 0.0439) (11.7233, 0.0589) knots 0 0 0 1 2 2 2
  line L116 (11.7233, 0.0589) -> (11.793, 0.2182)
  line L117 (11.793, 0.2182) -> (11.8826, 0.2182)
  line L118 (11.8826, 0.2182) -> (11.8826, -0.3742)
  line L119 (11.8826, -0.3742) -> (11.793, -0.3742)
  line L120 (11.793, 1.8642) -> (11.7316, 2.0334)
  spline S23 degree 2 poles (11.7316, 2.0334) (11.7233, 2.0517) (11.7018, 2.0732) (11.6785, 2.0732) knots 0 0 0 1 2 2 2
  line L121 (11.6785, 2.0732) -> (10.5834, 2.0732)
  spline S24 degree 2 poles (10.5834, 2.0732) (10.5618, 2.0732) (10.5386, 2.0484) (10.5336, 2.0334) knots 0 0 0 1 2 2 2
  line L122 (10.5336, 2.0334) -> (10.4722, 1.8642)
  line L123 (10.4722, 1.8642) -> (10.3826, 1.8642)
  line L124 (10.3826, 1.8642) -> (10.3826, 2.6274)
  line L125 (10.3826, 2.6274) -> (10.4722, 2.6274)
  line L126 (10.4722, 2.6274) -> (10.5336, 2.4599)
  spline S25 degree 2 poles (10.5336, 2.4599) (10.5386, 2.4433) (10.5618, 2.4184) (10.5834, 2.4184) knots 0 0 0 1 2 2 2
  line L127 (10.5834, 2.4184) -> (11.6785, 2.4184)
  spline S26 degree 2 poles (11.6785, 2.4184) (11.7018, 2.4184) (11.725, 2.4416) (11.7316, 2.4599) knots 0 0 0 1 2 2 2
  line L128 (11.7316, 2.4599) -> (11.793, 2.6274)
  line L129 (11.793, 2.6274) -> (11.8826, 2.6274)
  line L130 (11.8826, 2.6274) -> (11.8826, 1.8642)
  line L131 (11.8826, 1.8642) -> (11.793, 1.8642)
  line L132 (11.793, 2.7403) -> (11.7466, 2.8714)
  spline S27 degree 2 poles (11.7466, 2.8714) (11.7383, 2.8913) (11.7051, 2.9245) (11.6868, 2.9394) knots 0 0 0 1 2 2 2
  line L133 (11.6868, 2.9394) -> (11.1625, 3.3575)
  line L134 (11.1625, 3.3575) -> (10.5718, 2.9493)
  spline S28 degree 2 poles (10.5718, 2.9493) (10.5552, 2.9377) (10.5237, 2.9029) (10.517, 2.8846) knots 0 0 0 1 2 2 2
  line L135 (10.517, 2.8846) -> (10.4722, 2.7602)
  line L136 (10.4722, 2.7602) -> (10.3826, 2.7602)
  line L137 (10.3826, 2.7602) -> (10.3826, 3.4637)
  line L138 (10.3826, 3.4637) -> (10.4722, 3.4637)
  line L139 (10.4722, 3.4637) -> (10.5336, 3.3227)
  line L140 (10.5336, 3.3227) -> (10.8339, 3.5284)
  line L141 (10.8339, 3.5284) -> (10.9567, 3.5932)
  line L142 (10.9567, 3.5932) -> (10.9567, 3.5998)
  line L143 (10.9567, 3.5998) -> (10.5419, 3.9134)
  line L144 (10.5419, 3.9134) -> (10.4722, 3.779)
  line L145 (10.4722, 3.779) -> (10.3826, 3.779)
  line L146 (10.3826, 3.779) -> (10.3826, 4.3)
  line L147 (10.3826, 4.3) -> (10.4722, 4.3)
  line L148 (10.4722, 4.3) -> (10.5187, 4.1805)
  spline S29 degree 2 poles (10.5187, 4.1805) (10.5253, 4.1656) (10.5585, 4.1291) (10.5751, 4.1142) knots 0 0 0 1 2 2 2
  line L149 (10.5751, 4.1142) -> (11.0895, 3.7093)
  line L150 (11.0895, 3.7093) -> (11.6918, 4.1274)
  spline S30 degree 2 poles (11.6918, 4.1274) (11.7101, 4.1407) (11.7416, 4.1739) (11.7482, 4.1922) knots 0 0 0 1 2 2 2
  line L151 (11.7482, 4.1922) -> (11.793, 4.3166)
  line L152 (11.793, 4.3166) -> (11.8826, 4.3166)
  line L153 (11.8826, 4.3166) -> (11.8826, 3.6147)
  line L154 (11.8826, 3.6147) -> (11.793, 3.6147)
  line L155 (11.793, 3.6147) -> (11.73, 3.7558)
  line L156 (11.73, 3.7558) -> (11.4147, 3.5384)
  line L157 (11.4147, 3.5384) -> (11.2936, 3.4737)
  line L158 (11.2936, 3.4737) -> (11.2936, 3.467)
  line L159 (11.2936, 3.467) -> (11.7233, 3.1385)
  line L160 (11.7233, 3.1385) -> (11.793, 3.2713)
  line L161 (11.793, 3.2713) -> (11.8826, 3.2713)
  line L162 (11.8826, 3.2713) -> (11.8826, 2.7403)
  line L163 (11.8826, 2.7403) -> (11.793, 2.7403)
  line L164 (11.793, 4.4294) -> (11.7316, 4.5904)
  spline S31 degree 2 poles (11.7316, 4.5904) (11.725, 4.607) (11.7018, 4.6302) (11.6785, 4.6302) knots 0 0 0 1 2 2 2
  line L165 (11.6785, 4.6302) -> (10.5834, 4.6302)
  spline S32 degree 2 poles (10.5834, 4.6302) (10.5618, 4.6302) (10.5386, 4.607) (10.5336, 4.5904) knots 0 0 0 1 2 2 2
  line L166 (10.5336, 4.5904) -> (10.4722, 4.4294)
  line L167 (10.4722, 4.4294) -> (10.3826, 4.4294)
  line L168 (10.3826, 4.4294) -> (10.3826, 5.732)
  line L169 (10.3826, 5.732) -> (10.8024, 5.732)
  line L170 (10.8024, 5.732) -> (10.8024, 5.5926)
  line L171 (10.8024, 5.5926) -> (10.5983, 5.5329)
  spline S33 degree 2 poles (10.5983, 5.5329) (10.5801, 5.5262) (10.5585, 5.5063) (10.5585, 5.4881) knots 0 0 0 1 2 2 2
  line L172 (10.5585, 5.4881) -> (10.5585, 4.9753)
  line L173 (10.5585, 4.9753) -> (11.0181, 4.9753)
  line L174 (11.0181, 4.9753) -> (11.0181, 5.2574)
  spline S34 degree 2 poles (11.0181, 5.2574) (11.0181, 5.2807) (10.9999, 5.2972) (10.98, 5.3022) knots 0 0 0 1 2 2 2
  line L175 (10.98, 5.3022) -> (10.8157, 5.3603)
  line L176 (10.8157, 5.3603) -> (10.8157, 5.4748)
  line L177 (10.8157, 5.4748) -> (11.3882, 5.4748)
  line L178 (11.3882, 5.4748) -> (11.3882, 5.3603)
  line L179 (11.3882, 5.3603) -> (11.2255, 5.3022)
  spline S35 degree 2 poles (11.2255, 5.3022) (11.2073, 5.2972) (11.1857, 5.2807) (11.1857, 5.2574) knots 0 0 0 1 2 2 2
  line L180 (11.1857, 5.2574) -> (11.1857, 4.9753)
  line L181 (11.1857, 4.9753) -> (11.7051, 4.9753)
  line L182 (11.7051, 4.9753) -> (11.7051, 5.5694)
  spline S36 degree 2 poles (11.7051, 5.5694) (11.7051, 5.5843) (11.6835, 5.6092) (11.6653, 5.6125) knots 0 0 0 1 2 2 2
  line L183 (11.6653, 5.6125) -> (11.4346, 5.6722)
  line L184 (11.4346, 5.6722) -> (11.4346, 5.8116)
  line L185 (11.4346, 5.8116) -> (11.8826, 5.8116)
  line L186 (11.8826, 5.8116) -> (11.8826, 4.4294)
  line L187 (11.8826, 4.4294) -> (11.793, 4.4294)
  line L188 (11.793, 6.0141) -> (11.7316, 6.175)
  spline S37 degree 2 poles (11.7316, 6.175) (11.7266, 6.1916) (11.7018, 6.2148) (11.6785, 6.2148) knots 0 0 0 1 2 2 2
  line L189 (11.6785, 6.2148) -> (10.5834, 6.2148)
  spline S38 degree 2 poles (10.5834, 6.2148) (10.5618, 6.2148) (10.5386, 6.1916) (10.5336, 6.175) knots 0 0 0 1 2 2 2
  line L190 (10.5336, 6.175) -> (10.4722, 6.0141)
  line L191 (10.4722, 6.0141) -> (10.3826, 6.0141)
  line L192 (10.3826, 6.0141) -> (10.3826, 6.7624)
  line L193 (10.3826, 6.7624) -> (10.4722, 6.7624)
  line L194 (10.4722, 6.7624) -> (10.5336, 6.6015)
  spline S39 degree 2 poles (10.5336, 6.6015) (10.5403, 6.5849) (10.5618, 6.56) (10.5834, 6.56) knots 0 0 0 1 2 2 2
  line L195 (10.5834, 6.56) -> (11.7051, 6.56)
  line L196 (11.7051, 6.56) -> (11.7051, 7.0578)
  spline S40 degree 2 poles (11.7051, 7.0578) (11.7051, 7.0661) (11.6984, 7.081) (11.6868, 7.0943) (11.6719, 7.1009) (11.6603, 7.1026) knots 0 0 0 1 2 3 4 4 4
  line L197 (11.6603, 7.1026) -> (11.3533, 7.1689)
  line L198 (11.3533, 7.1689) -> (11.3533, 7.31)
  line L199 (11.3533, 7.31) -> (11.8826, 7.31)
  line L200 (11.8826, 7.31) -> (11.8826, 6.0141)
  line L201 (11.8826, 6.0141) -> (11.793, 6.0141)
  line L202 (13.9549, -1.5138) -> (13.1134, -1.901)
  line L203 (13.1134, -1.901) -> (13.7817, -1.901)
  spline S41 degree 2 poles (13.7817, -1.901) (13.874, -1.901) (13.8969, -1.8814) knots 0 0 0 1 1 1
  spline S42 degree 2 poles (13.8969, -1.8814) (13.9279, -1.8536) (13.9279, -1.7948) knots 0 0 0 1 1 1
  line L204 (13.9279, -1.7948) -> (13.9279, -1.7597)
  line L205 (13.9279, -1.7597) -> (13.9549, -1.7597)
  line L206 (13.9549, -1.7597) -> (13.9549, -2.1069)
  line L207 (13.9549, -2.1069) -> (13.9279, -2.1069)
  line L208 (13.9279, -2.1069) -> (13.9279, -2.0718)
  spline S43 degree 2 poles (13.9279, -2.0718) (13.9279, -2.008) (13.8895, -1.9819) knots 0 0 0 1 1 1
  spline S44 degree 2 poles (13.8895, -1.9819) (13.8658, -1.9656) (13.7817, -1.9656) knots 0 0 0 1 1 1
  line L209 (13.7817, -1.9656) -> (13.1281, -1.9656)
  spline S45 degree 2 poles (13.1281, -1.9656) (13.0619, -1.9656) (13.0317, -1.9803) knots 0 0 0 1 1 1
  spline S46 degree 2 poles (13.0317, -1.9803) (13.0105, -1.9909) (12.9819, -2.0456) (12.9819, -2.1069) knots 0 0 0 1 2 2 2
  line L210 (12.9819, -2.1069) -> (12.9549, -2.1069)
  line L211 (12.9549, -2.1069) -> (12.9549, -1.8234)
  line L212 (12.9549, -1.8234) -> (13.7376, -1.4606)
  line L213 (13.7376, -1.4606) -> (12.9549, -1.1028)
  line L214 (12.9549, -1.1028) -> (12.9549, -0.8209)
  line L215 (12.9549, -0.8209) -> (12.9819, -0.8209)
  line L216 (12.9819, -0.8209) -> (12.9819, -0.8553)
  spline S47 degree 2 poles (12.9819, -0.8553) (12.9819, -0.9198) (13.0203, -0.9459) knots 0 0 0 1 1 1
  spline S48 degree 2 poles (13.0203, -0.9459) (13.0439, -0.9623) (13.1281, -0.9623) knots 0 0 0 1 1 1
  line L217 (13.1281, -0.9623) -> (13.7817, -0.9623)
  spline S49 degree 2 poles (13.7817, -0.9623) (13.874, -0.9623) (13.8969, -0.9419) knots 0 0 0 1 1 1
  spline S50 degree 2 poles (13.8969, -0.9419) (13.9279, -0.9141) (13.9279, -0.8553) knots 0 0 0 1 1 1
  line L218 (13.9279, -0.8553) -> (13.9279, -0.8209)
  line L219 (13.9279, -0.8209) -> (13.9549, -0.8209)
  line L220 (13.9549, -0.8209) -> (13.9549, -1.245)
  line L221 (13.9549, -1.245) -> (13.9279, -1.245)
  line L222 (13.9279, -1.245) -> (13.9279, -1.2098)
  spline S51 degree 2 poles (13.9279, -1.2098) (13.9279, -1.1453) (13.8895, -1.12) knots 0 0 0 1 1 1
  spline S52 degree 2 poles (13.8895, -1.12) (13.8658, -1.1036) (13.7817, -1.1036) knots 0 0 0 1 1 1
  line L223 (13.7817, -1.1036) -> (13.1134, -1.1036)
  line L224 (13.1134, -1.1036) -> (13.9549, -1.4892)
  line L225 (13.9549, -1.4892) -> (13.9549, -1.5138)
  line L226 (13.401, -0.1731) -> (13.7212, 0.0418)
  spline S53 degree 2 poles (13.7212, 0.0418) (13.8544, 0.1309) (13.9239, 0.2175) (13.9279, 0.2836) knots 0 0 0 1 2 2 2
  line L227 (13.9279, 0.2836) -> (13.9549, 0.2836)
  line L228 (13.9549, 0.2836) -> (13.9549, -0.1453)
  line L229 (13.9549, -0.1453) -> (13.9279, -0.1453)
  spline S54 degree 2 poles (13.9279, -0.1453) (13.9271, -0.1028) (13.9189, -0.0824) knots 0 0 0 1 1 1
  spline S55 degree 2 poles (13.9189, -0.0824) (13.9124, -0.0669) (13.8855, -0.0464) (13.8707, -0.0464) knots 0 0 0 1 2 2 2
  spline S56 degree 2 poles (13.8707, -0.0464) (13.8544, -0.0464) (13.8373, -0.053) knots 0 0 0 1 1 1
  spline S57 degree 2 poles (13.8373, -0.053) (13.825, -0.0587) (13.7719, -0.0938) knots 0 0 0 1 1 1
  line L230 (13.7719, -0.0938) -> (13.517, -0.2638)
  line L231 (13.517, -0.2638) -> (13.7841, -0.4729)
  spline S58 degree 2 poles (13.7841, -0.4729) (13.8266, -0.5056) (13.8552, -0.5195) (13.8707, -0.5195) knots 0 0 0 1 2 2 2
  spline S59 degree 2 poles (13.8707, -0.5195) (13.8944, -0.5195) (13.9255, -0.4794) (13.9279, -0.4231) knots 0 0 0 1 2 2 2
  line L232 (13.9279, -0.4231) -> (13.9549, -0.4231)
  line L233 (13.9549, -0.4231) -> (13.9549, -0.7785)
  line L234 (13.9549, -0.7785) -> (13.9279, -0.7785)
  spline S60 degree 2 poles (13.9279, -0.7785) (13.9239, -0.7401) (13.9124, -0.7131) knots 0 0 0 1 1 1
  spline S61 degree 2 poles (13.9124, -0.7131) (13.8928, -0.6673) (13.8283, -0.5848) (13.7613, -0.5317) knots 0 0 0 1 2 2 2
  line L235 (13.7613, -0.5317) -> (13.4639, -0.2997)
  line L236 (13.4639, -0.2997) -> (13.1747, -0.4925)
  spline S62 degree 2 poles (13.1747, -0.4925) (13.057, -0.5726) (12.9843, -0.6853) (12.9819, -0.758) knots 0 0 0 1 2 2 2
  line L237 (12.9819, -0.758) -> (12.9549, -0.758)
  line L238 (12.9549, -0.758) -> (12.9549, -0.2948)
  line L239 (12.9549, -0.2948) -> (12.9819, -0.2948)
  spline S63 degree 2 poles (12.9819, -0.2948) (12.9843, -0.3544) (13.0178, -0.3977) (13.0382, -0.3977) knots 0 0 0 1 2 2 2
  spline S64 degree 2 poles (13.0382, -0.3977) (13.066, -0.3977) (13.1183, -0.3626) knots 0 0 0 1 1 1
  line L240 (13.1183, -0.3626) -> (13.3479, -0.2082)
  line L241 (13.3479, -0.2082) -> (13.1224, -0.0317)
  spline S65 degree 2 poles (13.1224, -0.0317) (13.0823, -0.0007) (13.0529, 0.0132) (13.0374, 0.0132) knots 0 0 0 1 2 2 2
  spline S66 degree 2 poles (13.0374, 0.0132) (13.0227, 0.0132) (13.0105, 0.0042) knots 0 0 0 1 1 1
  spline S67 degree 2 poles (13.0105, 0.0042) (12.9949, -0.0072) (12.9827, -0.0407) (12.9819, -0.0938) knots 0 0 0 1 2 2 2
  line L242 (12.9819, -0.0938) -> (12.9549, -0.0938)
  line L243 (12.9549, -0.0938) -> (12.9549, 0.2608)
  line L244 (12.9549, 0.2608) -> (12.9819, 0.2608)
  spline S68 degree 2 poles (12.9819, 0.2608) (12.9843, 0.2191) (12.9949, 0.1921) knots 0 0 0 1 1 1
  spline S69 degree 2 poles (12.9949, 0.1921) (13.0121, 0.1521) (13.0693, 0.0859) (13.1469, 0.0255) knots 0 0 0 1 2 2 2
  line L245 (13.1469, 0.0255) -> (13.401, -0.1731)
  line L246 (13.5603, 0.3629) -> (13.5603, 0.7452)
  line L247 (13.5603, 0.7452) -> (13.6714, 0.7452)
  line L248 (13.6714, 0.7452) -> (13.6714, 0.3629)
  line L249 (13.6714, 0.3629) -> (13.5603, 0.3629)
  line L250 (12.9345, 1.483) -> (12.9614, 1.483)
  spline S70 degree 2 poles (12.9614, 1.483) (12.9712, 1.3858) (13.0292, 1.2616) (13.1485, 1.1415) (13.2956, 1.0622) (13.3969, 1.0353) knots 0 0 0 1 2 3 4 4 4
  spline S71 degree 2 poles (13.3969, 1.0353) (13.3234, 1.1423) (13.3234, 1.2493) knots 0 0 0 1 1 1
  spline S72 degree 2 poles (13.3234, 1.2493) (13.3234, 1.3514) (13.4884, 1.5026) (13.6183, 1.5026) knots 0 0 0 1 2 2 2
  spline S73 degree 2 poles (13.6183, 1.5026) (13.7433, 1.5026) (13.8471, 1.4266) knots 0 0 0 1 1 1
  spline S74 degree 2 poles (13.8471, 1.4266) (13.9721, 1.3351) (13.9721, 1.184) knots 0 0 0 1 1 1
  spline S75 degree 2 poles (13.9721, 1.184) (13.9721, 1.0818) (13.9042, 1.0099) knots 0 0 0 1 1 1
  spline S76 degree 2 poles (13.9042, 1.0099) (13.7727, 0.8694) (13.5619, 0.8694) knots 0 0 0 1 1 1
  spline S77 degree 2 poles (13.5619, 0.8694) (13.4279, 0.8694) (13.1861, 0.9773) (12.999, 1.1774) (12.9345, 1.3612) (12.9345, 1.4405) knots 0 0 0 1 2 3 4 4 4
  line L251 (12.9345, 1.4405) -> (12.9345, 1.483)
  spline S78 degree 2 poles (13.4508, 1.023) (13.5497, 1.0099) (13.6109, 1.0099) knots 0 0 0 1 1 1
  spline S79 degree 2 poles (13.6109, 1.0099) (13.6812, 1.0099) (13.8471, 1.0622) (13.8961, 1.1137) knots 0 0 0 1 2 2 2
  spline S80 degree 2 poles (13.8961, 1.1137) (13.9304, 1.1521) (13.9304, 1.206) knots 0 0 0 1 1 1
  spline S81 degree 2 poles (13.9304, 1.206) (13.9304, 1.2697) (13.8095, 1.371) (13.6975, 1.371) knots 0 0 0 1 2 2 2
  spline S82 degree 2 poles (13.6975, 1.371) (13.5717, 1.371) (13.3879, 1.2706) (13.3879, 1.1782) knots 0 0 0 1 2 2 2
  spline S83 degree 2 poles (13.3879, 1.1782) (13.3879, 1.1505) (13.4116, 1.0859) (13.4508, 1.023) knots 0 0 0 1 2 2 2
  line L252 (13.5864, 2.264) -> (13.691, 2.264)
  line L253 (13.691, 2.264) -> (13.691, 2.13)
  line L254 (13.691, 2.13) -> (13.9549, 2.13)
  line L255 (13.9549, 2.13) -> (13.9549, 2.0083)
  line L256 (13.9549, 2.0083) -> (13.691, 2.0083)
  line L257 (13.691, 2.0083) -> (13.691, 1.5843)
  line L258 (13.691, 1.5843) -> (13.5971, 1.5843)
  line L259 (13.5971, 1.5843) -> (12.9345, 2.0492)
  line L260 (12.9345, 2.0492) -> (12.9345, 2.13)
  line L261 (12.9345, 2.13) -> (13.5864, 2.13)
  line L262 (13.5864, 2.13) -> (13.5864, 2.264)
  line L263 (13.5864, 2.0083) -> (13.0897, 2.0083)
  line L264 (13.0897, 2.0083) -> (13.5864, 1.657)
  line L265 (13.5864, 1.657) -> (13.5864, 2.0083)
  point P0 (0, 0)
  dimension "d0" = 61.1
  dimension "d1" = 40.2
  dimension "d2" = 10
  dimension "d3" = 13
  dimension "d4" = 28
  dimension "d5" = 55.5
  dimension "d6" = 29
  dimension "d9" = 4
  dimension "d10" = 2.8
  dimension "d13" = 34.6
  dimension "d16" = 22
  dimension "d20" = 2.8
  dimension "d23" = 22
  dimension "d24" = 11
  dimension "d25" = 8
  constraints: 2 other